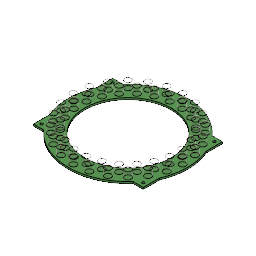
ring-light-67mm (Autodesk Fusion 360 design; units mm, degrees)
Autodesk Fusion 360 part; units mm, degrees
note: some values were not read from the file. Set by a fixed rule: which sketch regions a step uses.
sketch "PCB Outline" plane through (0, 0, 0) normal (0, 1, 0) x (1, 0, 0)
  circle A0 centre (0, 0) radius 33.9
  circle A1 centre (0, 0) radius 47
  line L0 (-40, 28) -> (40, 28)
  line L1 (40, 28) -> (40, -28)
  line L2 (40, -28) -> (-40, -28)
  line L3 (-40, -28) -> (-40, 28)
  line L4 (0, 28) -> (0, 0) construction
  line L5 (0, 0) -> (-40, 0) construction
  line L6 (-43.25, 31.25) -> (43.25, 31.25)
  line L7 (43.25, 31.25) -> (43.25, -31.25)
  line L8 (43.25, -31.25) -> (-43.25, -31.25)
  line L9 (-43.25, -31.25) -> (-43.25, 31.25)
  line L10 (0, 31.25) -> (0, 0) construction
  line L11 (0, 0) -> (-43.25, 0) construction
  circle A2 centre (-40, 28) radius 1
  circle A3 centre (40, 28) radius 1
  circle A4 centre (40, -28) radius 1
  circle A5 centre (-40, -28) radius 1
  dimension "d1" = 67.8
  dimension "d2" = 94
  dimension "d3" = 80
  dimension "d4" = 56
  dimension "d5" = 86.5
  dimension "d6" = 62.5
  dimension "d7" = 2
  measures "d1" diameter of A0
  measures "d2" diameter of A1
  measures "d7" diameter of A2
extrude "Extrude1" add sketch "PCB Outline" along normal blind 1.5 contours A0 A1 L0 L1 L2 | A0 A1 L0 L6 | A0 A1 L2 L8 | A0 A1 L6 | A0 A1 L0 L6 | A0 A1 L0 L2 L3 | A1 L0 L1 A3 | A1 L0 L1 L6 L7 A3 | A0 A1 L8 | A1 L1 L2 L7 L8 A4 | A1 L1 L2 A4 | A0 A1 L2 L8 | A1 L0 L3 L6 L9 A2 | A1 L0 L3 A2 | A1 L1 L7 | A1 L2 L3 A5 | A1 L2 L3 L8 L9 A5 | A1 L3 L9 | A1 L7 | A1 L9 makes body 1
sketch "LEDs" plane through (0, 1.5, 0) normal (0, 1, 0) x (-1, 0, 0)
  circle A0 centre (-40, 28) radius 1
  circle A1 centre (40, 28) radius 1
  circle A2 centre (40, -28) radius 1
  circle A3 centre (0, 0) radius 33.9
  circle A4 centre (-40, -28) radius 1
  arc A5 (35.1061, 31.25) -> (-35.1061, 31.25) centre (0, 0) ccw
  line L0 (-35.1061, 31.25) -> (-43.25, 31.25)
  line L1 (-43.25, 31.25) -> (-43.25, 18.3967)
  arc A6 (-43.25, 18.3967) -> (-43.25, -18.3967) centre (0, 0) ccw
  line L2 (-43.25, -18.3967) -> (-43.25, -31.25)
  line L3 (-43.25, -31.25) -> (-35.1061, -31.25)
  arc A7 (-35.1061, -31.25) -> (35.1061, -31.25) centre (0, 0) ccw
  line L4 (35.1061, -31.25) -> (43.25, -31.25)
  line L5 (43.25, -31.25) -> (43.25, -18.3967)
  arc A8 (43.25, -18.3967) -> (43.25, 18.3967) centre (0, 0) ccw
  line L6 (43.25, 18.3967) -> (43.25, 31.25)
  line L7 (43.25, 31.25) -> (35.1061, 31.25)
  circle A9 centre (0, 0) radius 38 construction
  circle A10 centre (0, 0) radius 43 construction
  line L8 (0, 0) -> (0, -43) construction
  circle A11 centre (0, -43) radius 2.5
  circle A12 centre (11.1292, -41.5348) radius 2.5
  circle A13 centre (21.5, -37.2391) radius 2.5
  circle A14 centre (30.4056, -30.4056) radius 2.5
  circle A15 centre (37.2391, -21.5) radius 2.5
  circle A16 centre (41.5348, -11.1292) radius 2.5
  circle A17 centre (43, 0) radius 2.5
  circle A18 centre (41.5348, 11.1292) radius 2.5
  circle A19 centre (37.2391, 21.5) radius 2.5
  circle A20 centre (30.4056, 30.4056) radius 2.5
  circle A21 centre (21.5, 37.2391) radius 2.5
  circle A22 centre (11.1292, 41.5348) radius 2.5
  circle A23 centre (0, 43) radius 2.5
  circle A24 centre (-11.1292, 41.5348) radius 2.5
  circle A25 centre (-21.5, 37.2391) radius 2.5
  circle A26 centre (-30.4056, 30.4056) radius 2.5
  circle A27 centre (-37.2391, 21.5) radius 2.5
  circle A28 centre (-41.5348, 11.1292) radius 2.5
  circle A29 centre (-43, 0) radius 2.5
  circle A30 centre (-41.5348, -11.1292) radius 2.5
  circle A31 centre (-37.2391, -21.5) radius 2.5
  circle A32 centre (-30.4056, -30.4056) radius 2.5
  circle A33 centre (-21.5, -37.2391) radius 2.5
  circle A34 centre (-11.1292, -41.5348) radius 2.5
  circle A35 centre (4.96, -37.6749) radius 2.5
  line L9 (0, 0) -> (4.96, -37.6749) construction
  circle A36 centre (14.542, -35.1074) radius 2.5
  circle A37 centre (23.1329, -30.1474) radius 2.5
  circle A38 centre (30.1474, -23.1329) radius 2.5
  circle A39 centre (35.1074, -14.542) radius 2.5
  circle A40 centre (37.6749, -4.96) radius 2.5
  circle A41 centre (37.6749, 4.96) radius 2.5
  circle A42 centre (35.1074, 14.542) radius 2.5
  circle A43 centre (30.1474, 23.1329) radius 2.5
  circle A44 centre (23.1329, 30.1474) radius 2.5
  circle A45 centre (14.542, 35.1074) radius 2.5
  circle A46 centre (4.96, 37.6749) radius 2.5
  circle A47 centre (-4.96, 37.6749) radius 2.5
  circle A48 centre (-14.542, 35.1074) radius 2.5
  circle A49 centre (-23.1329, 30.1474) radius 2.5
  circle A50 centre (-30.1474, 23.1329) radius 2.5
  circle A51 centre (-35.1074, 14.542) radius 2.5
  circle A52 centre (-37.6749, 4.96) radius 2.5
  circle A53 centre (-37.6749, -4.96) radius 2.5
  circle A54 centre (-35.1074, -14.542) radius 2.5
  circle A55 centre (-30.1474, -23.1329) radius 2.5
  circle A56 centre (-23.1329, -30.1474) radius 2.5
  circle A57 centre (-14.542, -35.1074) radius 2.5
  circle A58 centre (-4.96, -37.6749) radius 2.5
  dimension "d10" = 76
  dimension "d11" = 86
  dimension "d12" = 5
  dimension "d14" = 360
  dimension "d15" = 7.5
  dimension "d17" = 360
  measures "d10" diameter of A9
  measures "d11" diameter of A10
  measures "d12" diameter of A11
  measures "d15" angle of L8 L9
extrude "Extrude2" add sketch "LEDs" along normal blind 8 separate body contours A11 | A12 | A13 | A14 | A15 | A16 | A17 | A18 | A19 | A20 | A21 | A22 | A23 | A24 | A25 | A26 | A27 | A28 | A29 | A30 | A31 | A32 | A33 | A34 | A35 | A36 | A37 | A38 | A39 | A40 | A41 | A42 | A43 | A44 | A45 | A46 | A47 | A48 | A49 | A50 | A51 | A52 | A53 | A54 | A55 | A56 | A57 | A58 makes body 2 at (-17.0389, 6.8333, -35.232) makes body 3 at (2.4631, 6.8333, -37.7995) makes body 4 at (20.636, 6.8333, -30.272) makes body 5 at (32.6105, 6.8333, -14.6666) makes body 6 at (35.178, 6.8333, 4.8354) makes body 7 at (27.6505, 6.8333, 23.0083) makes body 8 at (12.0451, 6.8333, 34.9828) makes body 9 at (-7.4569, 6.8333, 37.5503) makes body 10 at (-25.6298, 6.8333, 30.0228) makes body 11 at (-37.6043, 6.8333, 14.4174) makes body 12 at (-40.1718, 6.8333, -5.0846) makes body 13 at (-32.6443, 6.8333, -23.2575) makes body 14 at (-39.736, 6.8333, -21.6246) makes body 15 at (-45.4969, 6.8333, -0.1246) makes body 16 at (-39.736, 6.8333, 21.3754) makes body 17 at (-23.9969, 6.8333, 37.1145) makes body 18 at (-2.4969, 6.8333, 42.8754) makes body 19 at (19.0031, 6.8333, 37.1145) makes body 20 at (34.7422, 6.8333, 21.3754) makes body 21 at (40.5031, 6.8333, -0.1246) makes body 22 at (34.7422, 6.8333, -21.6246) makes body 23 at (19.0031, 6.8333, -37.3637) makes body 24 at (-2.4969, 6.8333, -43.1246) makes body 25 at (-23.9969, 6.8333, -37.3637) makes body 26 at (-13.6261, 6.8333, -41.6594) makes body 27 at (8.6323, 6.8333, -41.6594) makes body 28 at (27.9087, 6.8333, -30.5302) makes body 29 at (39.0379, 6.8333, -11.2538) makes body 30 at (39.0379, 6.8333, 11.0046) makes body 31 at (27.9087, 6.8333, 30.281) makes body 32 at (2.4631, 6.8333, 37.5503) makes body 33 at (-13.6261, 6.8333, 41.4102) makes body 34 at (-32.9025, 6.8333, 30.281) makes body 35 at (-40.1718, 6.8333, 4.8354) makes body 36 at (-37.6043, 6.8333, -14.6666) makes body 37 at (-32.9025, 6.8333, -30.5302) makes body 38 at (-44.0317, 6.8333, -11.2538) makes body 39 at (-44.0317, 6.8333, 11.0046) makes body 40 at (-32.6443, 6.8333, 23.0083) makes body 41 at (-17.0389, 6.8333, 34.9828) makes body 42 at (8.6323, 6.8333, 41.4102) makes body 43 at (20.636, 6.8333, 30.0228) makes body 44 at (32.6105, 6.8333, 14.4174) makes body 45 at (35.178, 6.8333, -5.0846) makes body 46 at (27.6505, 6.8333, -23.2575) makes body 47 at (12.0451, 6.8333, -35.232) makes body 48 at (-7.4569, 6.8333, -37.7995) makes body 49 at (-25.6298, 6.8333, -30.272)
fillet "Fillet1" radius 2.5 48 edges at (25.4638, 9.5, 29.2434) (7.2908, 9.5, 36.7709) (-35.3441, 9.5, -5.864) (16.8728, 9.5, 34.2034) (37.4382, 9.5, 13.6379) (37.4382, 9.5, -15.446) (-8.7984, 9.5, 40.6308) (43.8656, 9.5, 10.2252) (-20.8021, 9.5, 29.2434) (23.8308, 9.5, 36.3351) (32.4782, 9.5, 22.2289) (13.46, 9.5, 40.6308) (32.7364, 9.5, 29.5016) (40.0057, 9.5, -5.864) (45.3308, 9.5, -0.904) (-35.3441, 9.5, 4.056) (-27.8166, 9.5, 22.2289) (-39.204, 9.5, 10.2252) (-40.6692, 9.5, -0.904) (43.8656, 9.5, -12.0333) (-2.6292, 9.5, 36.7709) (-19.1692, 9.5, 36.3351) (39.5699, 9.5, -22.404) (23.8308, 9.5, -38.1431) (16.8728, 9.5, -36.0115) (-20.8021, 9.5, -31.0515) (39.5699, 9.5, 20.596) (7.2908, 9.5, -38.5789) (-28.0748, 9.5, -31.3096) (25.4638, 9.5, -31.0515) (-19.1692, 9.5, -38.1431) (32.7364, 9.5, -31.3096) (-32.7766, 9.5, -15.446) (2.3308, 9.5, 42.096) (-8.7984, 9.5, -42.4388) (13.46, 9.5, -42.4388) (-12.2112, 9.5, 34.2034) (-34.9083, 9.5, -22.404) (-34.9083, 9.5, 20.596) (32.4782, 9.5, -24.037) (-2.6292, 9.5, -38.5789) (-12.2112, 9.5, -36.0115) (-32.7766, 9.5, 13.6379) (40.0057, 9.5, 4.056) (2.3308, 9.5, -43.904) (-28.0748, 9.5, 29.5016) (-39.204, 9.5, -12.0333) (-27.8166, 9.5, -24.037) on bodies 2 3 4 5 6 7 8 9 10 11 12 13 14 15 16 17 18 19 20 21 22 23 24 25 26 27 28 29 30 31 32 33 34 35 36 37 38 39 40 41 42 43 44 45 46 47 48 49
equation "d15 = ( 360 / 24 / 2 ) * 1 deg"
named bodies: "PCB"
